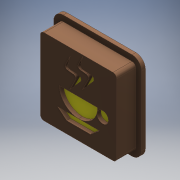
# Autodesk Inventor part: button3
Saved by Autodesk Inventor 2016 (Build 200138000, 138)
## iProperties
Created: 2017-11-06
Part Number: button3
Material: Bronze, Soft Tin
Document SubType Name: Modeling
Designer: Davide
Density: 8.874 g/cm^3
Appearance: Bronze - Satin
Author: Davide
Autodesk Inventor part; units mm, degrees
ref_plane "YZ Plane" through (0, 0, 0) normal (1, 0, 0) x (0, 1, 0)
ref_plane "XZ Plane" through (0, 0, 0) normal (0, 1, 0) x (-1, 0, 0)
ref_plane "XY Plane" through (0, 0, 0) normal (0, 0, 1) x (1, 0, 0)
sketch "Sketch1" plane through (0, 0, 0) normal (0, 1, 0) x (-1, 0, 0)
  line L0 (9, -10) -> (-9, -10)
  line L1 (-10, -9) -> (-10, 9)
  line L2 (-9, 10) -> (9, 10)
  line L3 (10, 9) -> (10, -9)
  line L4 (10, 10) -> (-10, -10) construction
  line L5 (10, -10) -> (-10, 10) construction
  arc A0 (10, 9) -> (9, 10) centre (9, 9) ccw
  arc A1 (9, -10) -> (10, -9) centre (9, -9) ccw
  arc A2 (-10, -9) -> (-9, -10) centre (-9, -9) ccw
  arc A3 (-9, 10) -> (-10, 9) centre (-9, 9) ccw
  point P0 (0, 0)
  point P1 (0, 0)
  dimension "d7" = 20
  dimension "d9" = 20
  dimension "d10" = 1
  constraints: 12 end point, 8 point on circle, 8 point on line, 8 tangent, 4 centre point, 3 equal radius, 2 parallel, 1 coincident, 1 horizontal, 1 midpoint, 1 perpendicular
  measures "d7" distance of L5.start L4.end
  measures "d9" distance of L4.end L5.end
  measures "d10" radius of A0
extrude "Extrusion1" add sketch "Sketch1" along normal blind 5
sketch "Sketch2" plane through (0, 5, 0) normal (0, 1, 0) x (1, 0, 0)
  line L0 (-10, 9) -> (-10, -9) projected
  arc A0 (-10, -9) -> (-9, -10) centre (-9, -9) ccw projected
  line L1 (-9, -10) -> (9, -10) projected
  arc A1 (9, -10) -> (10, -9) centre (9, -9) ccw projected
  line L2 (10, -9) -> (10, 9) projected
  arc A2 (10, 9) -> (9, 10) centre (9, 9) ccw projected
  line L3 (9, 10) -> (-9, 10) projected
  arc A3 (-9, 10) -> (-10, 9) centre (-9, 9) ccw projected
  line L4 (9, -11.5) -> (-9, -11.5)
  arc A4 (-11.5, -9) -> (-9, -11.5) centre (-9, -9) ccw
  line L5 (-11.5, -9) -> (-11.5, 9)
  arc A5 (-9, 11.5) -> (-11.5, 9) centre (-9, 9) ccw
  line L6 (-9, 11.5) -> (9, 11.5)
  arc A6 (11.5, 9) -> (9, 11.5) centre (9, 9) ccw
  line L7 (11.5, 9) -> (11.5, -9)
  arc A7 (9, -11.5) -> (11.5, -9) centre (9, -9) ccw
  circle A8 centre (0, 0) radius 2.75
  dimension "d16" = 1.5
  dimension "d19" = 5.5
  constraints: 8 end point, 8 point on circle, 5 centre point, 1 coincident, 7 other
  measures "d16" distance between parallel lines of L1 L4
  measures "d19" diameter of A8
extrude "Extrusion3" add sketch "Sketch2" along normal blind 1 contours A3 L3 A2 L2 A1 L1 A0 L0 | L4 A4 L5 A5 L6 A6 L7 A7
sketch "Sketch3" plane through (0, 0, 0) normal (0, -1, 0) x (1, 0, 0)
  line L0 (-3.1165, -7) -> (3.1165, -7)
  line L1 (3.1165, -7) -> (5.5, -5)
  line L2 (5.5, -5) -> (-5.5, -5)
  line L3 (-5.5, -5) -> (-3.1165, -7)
  line L4 (0, 0) -> (0, -4.6532) construction
  arc A0 (-5, 0) -> (5, 0) centre (0, 0) ccw
  circle A1 centre (6.3246, -1.5) radius 1.5
  line L5 (-5, 0) -> (5, 0)
  line L6 (-2.2003, 8.0155) -> (-3.4413, 5.57)
  line L7 (-2.9242, 4.5949) -> (-1.3286, 4.3927)
  line L8 (-0.8115, 3.4176) -> (-2.3458, 0.3942)
  line L9 (-2.2003, 8.0155) -> (-2.8111, 5.8955)
  line L10 (-2.2229, 5.0363) -> (0.0906, 4.8285)
  line L11 (0.5397, 3.7134) -> (-2.3458, 0.3942)
  arc A2 (-2.8111, 5.8955) -> (-2.2229, 5.0363) centre (-2.1625, 5.7086) ccw
  arc A3 (0.5397, 3.7134) -> (0.0906, 4.8285) centre (0.0303, 4.1562) ccw
  arc A4 (-0.8115, 3.4176) -> (-1.3286, 4.3927) centre (-1.4135, 3.723) ccw
  arc A5 (-3.4413, 5.57) -> (-2.9242, 4.5949) centre (-2.8393, 5.2646) ccw
  line L12 (1.1412, 9.7016) -> (-0.0998, 7.2561)
  line L13 (0.4173, 6.281) -> (2.0129, 6.0788)
  line L14 (2.53, 5.1037) -> (0.9957, 2.0803)
  line L15 (1.1412, 9.7016) -> (0.5304, 7.5816)
  line L16 (1.1186, 6.7224) -> (3.4321, 6.5146)
  line L17 (3.8812, 5.3995) -> (0.9957, 2.0803)
  arc A6 (0.5304, 7.5816) -> (1.1186, 6.7224) centre (1.179, 7.3947) ccw
  arc A7 (3.8812, 5.3995) -> (3.4321, 6.5146) centre (3.3717, 5.8423) ccw
  arc A8 (2.53, 5.1037) -> (2.0129, 6.0788) centre (1.928, 5.4091) ccw
  arc A9 (-0.0998, 7.2561) -> (0.4173, 6.281) centre (0.5022, 6.9507) ccw
  point P0 (0, -7)
  point P1 (0, -5)
  dimension "d68" = 10
  dimension "d69" = 11
  dimension "d70" = 2
  dimension "d71" = 100
  dimension "d72" = 3
  dimension "d73" = 0.675
  dimension "d74" = 0.675
  constraints: 36 end point, 19 tangent, 18 point on circle, 10 centre point, 6 equal radius, 3 midpoint, 3 parallel, 2 horizontal, 2 point on line, 1 coincident, 1 vertical, 1 other
  measures "d68" diameter of A0
  measures "d69" distance of L1.end L2.end
  measures "d70" distance between parallel lines of L0 L2
  measures "d71" angle of L1 L3
  measures "d72" diameter of A1
  measures "d73" radius of A2
  measures "d74" radius of A6
extrude "Extrusion7" cut sketch "Sketch3" against normal blind 1
hole "Hole1" at (0, 5, 0) direction (0, -1, 0) diameter 5.5 depth 3
equation "\"d7\" = button_side"
equation "\"d9\" = d7"
equation "\"d68\" = 0.5 * button_side"
equation "\"d69\" = 1.1 * d68"
equation "\"d70\" = 0.2 * d68"
equation "\"d72\" = 0.3 * d68"
equation "\"d0\" = 122"
equation "\"d1\" = 77"
equation "\"d4\" = 19"
equation "\"d5\" = 1"
equation "\"d8\" = 25"
equation "\"d13\" = 1.5"
equation "\"d14\" = 0"
equation "\"d15\" = 2"
equation "\"d30\" = 3.1"
equation "\"d31\" = 3"
equation "\"d33\" = 3"
equation "\"d34\" = 2"
equation "\"d36\" = 3"
equation "\"d38\" = 90deg"
equation "\"d39\" = 8"
equation "\"d40\" = 118deg"
equation "\"d44\" = 0"
equation "\"d45\" = 1.2"
equation "\"d46\" = 2"
equation "\"d47\" = 0"
equation "\"d50\" = 25"
equation "\"button_side\" = 20"
equation "\"d3\" = 1.01 * button_side"
equation "\"d2\" = d3"
body "Solid1"
